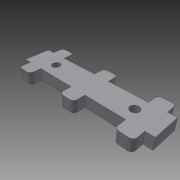
# Autodesk Inventor part: rope_mount_holder
Saved by Autodesk Inventor 2014 (Build 180170000, 170)
## iProperties
Created: 2013-12-08
Part Number: rope_mount_holder
Material: Generic
Document SubType Name: Modeling
Designer: buben
Density: 1 g/cm^3
Appearance: Default
Author: buben
Subject: Laser Cutted
Autodesk Inventor part; units mm, degrees
ref_plane "YZ Plane" through (0, 0, 0) normal (1, 0, 0) x (0, 1, 0)
ref_plane "XZ Plane" through (0, 0, 0) normal (0, 1, 0) x (-1, 0, 0)
ref_plane "XY Plane" through (0, 0, 0) normal (0, 0, 1) x (1, 0, 0)
sketch "Sketch1" plane through (0, 0, 0) normal (0, 0, 1) x (1, 0, 0)
  line L0 (0, 0) -> (72, 0)
  line L1 (72, 0) -> (72, 13.5)
  line L2 (72, 13.5) -> (0, 13.5)
  line L3 (0, 13.5) -> (0, 0)
  dimension "d0" = 13.5
  dimension "d1" = 72
  constraints: 8 end point, 2 parallel, 1 horizontal, 1 perpendicular
  measures "d0" distance of L2.end L0.start
  measures "d1" distance of L0.start L0.end
extrude "Extrusion1" add sketch "Sketch1" along normal blind 6
sketch "Sketch2" plane through (0, 0, 6) normal (0, 0, 1) x (1, 0, 0)
  line L0 (0, 0) -> (72, 0) projected
  line L1 (72, 0) -> (72, 13.5) projected
  line L2 (72, 13.5) -> (0, 13.5) projected
  line L3 (4, 13.5) -> (12, 13.5)
  line L4 (12, 13.5) -> (12, 17.5)
  line L5 (10, 19.5) -> (6, 19.5)
  line L6 (4, 17.5) -> (4, 13.5)
  line L7 (32, 13.5) -> (40, 13.5)
  line L8 (40, 13.5) -> (40, 17.5)
  line L9 (38, 19.5) -> (34, 19.5)
  line L10 (32, 17.5) -> (32, 13.5)
  line L11 (60, 13.5) -> (68, 13.5)
  line L12 (68, 13.5) -> (68, 17.5)
  line L13 (66, 19.5) -> (62, 19.5)
  line L14 (60, 17.5) -> (60, 13.5)
  line L15 (4, 0) -> (12, 0)
  line L16 (12, 0) -> (12, -4)
  line L17 (10, -6) -> (6, -6)
  line L18 (4, -4) -> (4, 0)
  line L19 (32, 0) -> (40, 0)
  line L20 (40, 0) -> (40, -4)
  line L21 (38, -6) -> (34, -6)
  line L22 (32, -4) -> (32, 0)
  line L23 (60, 0) -> (68, 0)
  line L24 (68, 0) -> (68, -4)
  line L25 (66, -6) -> (62, -6)
  line L26 (60, -4) -> (60, 0)
  arc A0 (6, 19.5) -> (4, 17.5) centre (6, 17.5) ccw
  arc A1 (12, 17.5) -> (10, 19.5) centre (10, 17.5) ccw
  arc A2 (34, 19.5) -> (32, 17.5) centre (34, 17.5) ccw
  arc A3 (40, 17.5) -> (38, 19.5) centre (38, 17.5) ccw
  arc A4 (62, 19.5) -> (60, 17.5) centre (62, 17.5) ccw
  arc A5 (68, 17.5) -> (66, 19.5) centre (66, 17.5) ccw
  arc A6 (4, -4) -> (6, -6) centre (6, -4) ccw
  arc A7 (10, -6) -> (12, -4) centre (10, -4) ccw
  arc A8 (32, -4) -> (34, -6) centre (34, -4) ccw
  arc A9 (38, -6) -> (40, -4) centre (38, -4) ccw
  arc A10 (60, -4) -> (62, -6) centre (62, -4) ccw
  arc A11 (66, -6) -> (68, -4) centre (66, -4) ccw
  line L27 (12, 15.5) -> (32, 15.5) construction
  line L28 (40, 15.5) -> (60, 15.5) construction
  point P0 (36, -6)
  point P1 (36, 0)
  dimension "d4" = 2
  dimension "d5" = 8
  dimension "d6" = 8
  dimension "d7" = 8
  dimension "d8" = 6
  dimension "d10" = 6
  dimension "d11" = 4
  constraints: 52 end point, 24 point on circle, 24 tangent, 12 centre point, 12 parallel, 11 collinear, 11 equal radius, 6 horizontal, 6 midpoint, 6 perpendicular, 6 point on line, 1 vertical alignment
  measures "d4" radius of A0
  measures "d5" distance between parallel lines of L4 L6
  measures "d6" distance between parallel lines of L8 L10
  measures "d7" distance between parallel lines of L12 L14
  measures "d8" distance between parallel lines of L3 L5
  measures "d10" distance between parallel lines of L15 L17
  measures "d11" distance between parallel lines of L1 L12
extrude "Extrusion2" add sketch "Sketch2" against normal blind 6
sketch "Sketch3" plane through (0, 0, 6) normal (0, 0, 1) x (1, 0, 0)
  line L0 (0, 13.5) -> (0, 0) projected
  circle A0 centre (58.715, 6.75) radius 2.25
  circle A1 centre (14.315, 6.75) radius 2.25
  point P0 (0, 6.75)
  dimension "d14" = 4.5
  dimension "d15" = 4.5
  dimension "d16" = 14.315
  dimension "d20" = 44.4
  constraints: 2 centre point, 2 horizontal alignment, 1 midpoint
  measures "d14" diameter of A0
  measures "d15" diameter of A1
  measures "d16" distance from line of L0 A1.centre
  measures "d20" distance of A0.centre A1.centre
extrude "Extrusion3" cut sketch "Sketch3" against normal through all
body "Solid1"
